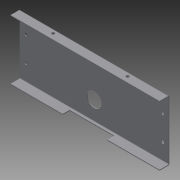
# Autodesk Inventor part: base_side_constr
Saved by Autodesk Inventor 2015 SP1 (Build 190203100, 203)
## iProperties
Created: 2015-04-20
Part Number: base_side_constr
Material: Ogólny
Document SubType Name: Konstrukcja blachowa
Designer: Marcin
Density: 1 g/cm^3
Sheet Metal Rule: Domyślny
Appearance: Domyślna
Flat Pattern Width: 7.80191 cm
Flat Pattern Length: 15.0111 cm
Flat Pattern Area: 117.115 cm^2
Sheet Metal Width: 78,019 mm
Sheet Metal Length: 150,111 mm
Sheet Metal Area: 11711,533 mm^2
Author: Marcin
Autodesk Inventor part; units mm, degrees
ref_plane "YZ Plane" through (0, 0, 0) normal (1, 0, 0) x (0, 1, 0)
ref_plane "XZ Plane" through (0, 0, 0) normal (0, 1, 0) x (-1, 0, 0)
ref_plane "XY Plane" through (0, 0, 0) normal (0, 0, 1) x (1, 0, 0)
ref_plane "Płaszczyzna konstrukcyjna1" through (0, 0, 0) normal (0, 0, 1) x (1, 0, 0)
sketch "Szkic2" plane through (0, 0, 0) normal (0, 0, 1) x (1, 0, 0)
  line L0 (0, 0.8) -> (-150.1111, 0.8)
  line L1 (-150.1111, 0) -> (-150.1111, 0.8)
  line L2 (0, 0) -> (-150.1111, 0)
  line L3 (0, 0) -> (0, 0.8)
  line L4 (-150.1111, 0) -> (0, 0)
  line L5 (0, 0) -> (0, 60)
  line L6 (0, 60) -> (-150.1111, 60)
  line L7 (-150.1111, 60) -> (-150.1111, 0)
  dimension "d0" = 60
  measures "d0" distance of L4.end L5.end
extrude "Płyta1" add sketch "Szkic2" along normal blind 0.8 contours L0 L7 L6 L5
sketch "Szkic3" plane through (-150.1111, 1.6, 0.8) normal (0, -1, 0) x (1, 0, 0)
  line L0 (150.1111, 0) -> (0, 0)
  line L1 (0, 0) -> (0, -10)
  line L2 (0, -10) -> (150.1111, -10)
  line L3 (150.1111, -10) -> (150.1111, 0)
  constraints: 6 end point, 1 horizontal, 1 perpendicular, 1 vertical
edge flange "Kołnierz1" height 10 angle 90 thickness 0.8 bend radius 0.8 thickness toward (0, -1, 0) relief straight relief width 0.8 relief depth 0.4 edges at (-75.0555, 0.8, 0) wall of the first edge with corners at (0, 1.6, 0.8) (-150.1111, 1.6, 0.8) (-150.1111, 1.6, -9.2) (0, 1.6, -9.2)
bend "Gięcie1"
corner "Narożnik1"
sketch "Szkic4" plane through (0, 60.8, -0.8) normal (0, 1, 0) x (-1, 0, 0)
  line L0 (150.1111, 0) -> (0, 0)
  line L1 (0, 0) -> (0, -8.4)
  line L2 (0, -8.4) -> (150.1111, -8.4)
  line L3 (150.1111, -8.4) -> (150.1111, 0)
  constraints: 6 end point, 1 horizontal, 1 perpendicular, 1 vertical
edge flange "Kołnierz2" height 10 angle 90 thickness 0.8 bend radius 0.8 thickness toward (0, 1, 0) relief straight relief width 0.8 relief depth 0.4 edges at (-75.0555, 60, 0) wall of the first edge with corners at (-150.1111, 60.8, -0.8) (0, 60.8, -0.8) (0, 60.8, -9.2) (-150.1111, 60.8, -9.2)
bend "Gięcie2"
corner "Narożnik2"
sketch "Szkic5" plane through (-150.1111, 0.8, -9.2) normal (0, -1, 0) x (1, 0, 0)
  line L0 (150.1111, 0) -> (0, 0) projected
  line L1 (0, 0) -> (150.1111, 0) construction
  line L2 (75.0555, 0) -> (75.0555, 31.3517) construction
  line L3 (52.5555, 0) -> (97.5555, 0)
  line L4 (97.5555, 0) -> (97.5555, 7)
  line L5 (97.5555, 7) -> (52.5555, 7)
  line L6 (52.5555, 7) -> (52.5555, 0)
  point P0 (150.1111, 9.2)
  dimension "d22" = 7
  dimension "d23" = 45
  constraints: 10 end point, 2 parallel, 1 horizontal, 1 midpoint, 1 perpendicular, 1 point on line, 1 vertical, 1 other
  measures "d22" distance of L3.end L4.end
  measures "d23" distance of L4.end L5.end
extrude "Wytnij1" cut sketch "Szkic5" against normal blind 0.8
sketch "Szkic6" plane through (-150.1111, 61.6, -9.2) normal (0, 1, 0) x (1, 0, 0)
  circle A0 centre (37.5555, -5.4) radius 1.5 projected
  circle A1 centre (112.5555, -5.4) radius 1.5 projected
  point P0 (150.1111, -9.2)
extrude "Wytnij2" cut sketch "Szkic6" against normal blind 0.8
sketch "Szkic7" plane through (0, 0, 0.8) normal (0, 0, 1) x (1, 0, 0)
  circle A0 centre (-143.9967, 43.1) radius 1.5 projected
  circle A1 centre (-143.9967, 18.1) radius 1.5 projected
  circle A2 centre (-6.1144, 18.1) radius 1.5 projected
  circle A3 centre (-6.1144, 43.1) radius 1.5 projected
  point P0 (0, 0)
extrude "Wytnij3" cut sketch "Szkic7" against normal blind 0.8
sketch "Szkic8" plane through (0, 0, 0.8) normal (0, 0, 1) x (1, 0, 0)
  circle A0 centre (-75.0555, 20.8) radius 7.5
  point P0 (0, 0)
  dimension "d30" = 15
  constraints: 1 centre point, 1 coincident, 1 other
  measures "d30" diameter of A0
extrude "Wytnij4" cut sketch "Szkic8" against normal blind 0.8
equation "\"d24\" = Grubość"
equation "\"d26\" = Grubość"
equation "\"d28\" = Grubość"
equation "\"d31\" = Grubość"
equation "\"d2\" = SzerokośćGięciaPodcięcia"
equation "\"d3\" = GłębokośćGięciaPodcięcia"
equation "\"d4\" = MinimalnaPozostałość"
equation "\"d5\" = PromieńGięcia"
equation "\"d8\" = PromieńGięcia"
equation "\"d9\" = RozmiarPodcięciaNarożnika"
equation "\"d10\" = Wielk_odstępu"
equation "\"d11\" = Rozmiar_promienia_Jacobiego"
equation "\"d12\" = SzerokośćGięciaPodcięcia"
equation "\"d13\" = GłębokośćGięciaPodcięcia"
equation "\"d14\" = MinimalnaPozostałość"
equation "\"d15\" = PromieńGięcia"
equation "\"d18\" = PromieńGięcia"
equation "\"d19\" = RozmiarPodcięciaNarożnika"
equation "\"d20\" = Wielk_odstępu"
equation "\"d21\" = Rozmiar_promienia_Jacobiego"
equation "\"PromieńGięcia\" = Grubość"
equation "\"SzerokośćGięciaPodcięcia\" = Grubość"
equation "\"GłębokośćGięciaPodcięcia\" = 0.5 * Grubość"
equation "\"RozmiarPodcięciaNarożnika\" = 4 * Grubość"
equation "\"MinimalnaPozostałość\" = 2 * Grubość"
equation "\"PromieńPrzejścia\" = PromieńGięcia"
equation "\"Rozmiar_promienia_Jacobiego\" = Grubość"
equation "\"Wielk_odstępu\" = Grubość"
equation "\"d1\" = PromieńGięcia"
equation "\"Grubość\" = 0.8"
